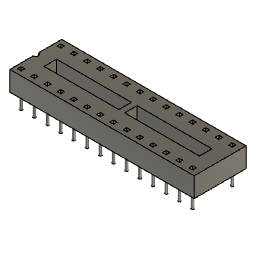
ICSocket_DIP28pin (Autodesk Fusion 360 design; units mm, degrees)
Autodesk Fusion 360 part; units mm, degrees
sketch "スケッチ1" plane through (0, 0, 0) normal (0, 0, 1) x (1, 0, 0)
  line L0 (-17.75, 5) -> (17.75, 5)
  line L1 (17.75, 5) -> (17.75, -5)
  line L2 (17.75, -5) -> (-17.75, -5)
  line L3 (-17.75, -5) -> (-17.75, 5)
  dimension "d1" = 35.5
  dimension "d2" = 10
  dimension "d3" = 17.75
  dimension "d4" = 5
  constraint horizontal L0
  constraint vertical L1
  constraint horizontal L2
  constraint vertical L3
  measures "d1" distance of L0.start L0.end
  measures "d2" distance of L0.start L2.end
  measures "d3" distance of origin L3
  measures "d4" distance of origin L0
extrude "押し出し1" add sketch "スケッチ1" along normal blind 3.8
sketch "スケッチ2" plane through (0, 0, 3.8) normal (0, 0, 1) x (-1, 0, 0)
  line L0 (17.75, 5) -> (-17.75, 5)
  line L1 (-17.75, 5) -> (-17.75, -5)
  line L2 (-17.75, -5) -> (17.75, -5)
  line L3 (17.75, -5) -> (17.75, 5)
  line L4 (-0.55, -1.2) -> (-14.95, -1.2)
  line L5 (-14.95, -1.2) -> (-14.95, 1.2)
  line L6 (-14.95, 1.2) -> (-0.55, 1.2)
  line L7 (-0.55, 1.2) -> (-0.55, -1.2)
  line L8 (14.95, -1.2) -> (0.55, -1.2)
  line L9 (0.55, -1.2) -> (0.55, 1.2)
  line L10 (0.55, 1.2) -> (14.95, 1.2)
  line L11 (14.95, 1.2) -> (14.95, -1.2)
  line L12 (0, -1.75) -> (0, -22.5)
  line L13 (17.11, 3.46) -> (16.41, 3.46)
  line L14 (16.41, 3.46) -> (16.41, 4.16)
  line L15 (16.41, 4.16) -> (17.11, 4.16)
  line L16 (17.11, 4.16) -> (17.11, 3.46)
  arc A0 (17.75, 0.5) -> (17.75, -0.5) centre (17.75, 0) ccw
  line L17 (17.75, 0) -> (17.75, 0.5) construction
  line L18 (17.75, 0) -> (17.75, -0.5) construction
  dimension "d7" = 14.4
  dimension "d8" = 2.4
  dimension "d9" = 3.8
  dimension "d10" = 2.8
  dimension "d11" = 14.4
  dimension "d12" = 2.4
  dimension "d17" = 0.7
  dimension "d18" = 0.7
  dimension "d19" = 3.46
  dimension "d20" = 0.64
  dimension "d38" = 0.5
  dimension "d39" = 180
  constraint horizontal L4
  constraint vertical L5
  constraint horizontal L6
  constraint vertical L7
  constraint horizontal L8
  constraint vertical L9
  constraint horizontal L10
  constraint vertical L11
  constraint collinear L6 L10
  constraint symmetric L7 L9 L12
  constraint horizontal L13
  constraint vertical L14
  constraint horizontal L15
  constraint vertical L16
  constraint midpoint L3 A0.centre
  measures "d7" distance of L4.start L4.end
  measures "d8" distance of L4.start L6.end
  measures "d9" distance of L0 L6
  measures "d10" distance of L1 L5
  measures "d11" distance of L8.start L8.end
  measures "d12" distance of L8.start L10.end
  measures "d17" distance of L13.start L13.end
  measures "d18" distance of L13.start L15.end
  measures "d19" distance of origin L13
  measures "d20" distance of L3 L16
  measures "d38" radius of A0
  measures "d39" angle of L17 L18
extrude "押し出し2" cut sketch "スケッチ2" against normal through all contours L3 A0 | L4 L5 L6 L7 | L8 L9 L10 L11
extrude "押し出し3" cut sketch "スケッチ2" against normal blind 3.5 contours L13 L14 L15 L16
pattern_linear "R パターン1" count 14 spacing 2.54 along (1, 0, 0) of "押し出し3"
mirror "ミラー1" about plane through (0, 0, 0) normal (0, 1, 0) of "押し出し3", "R パターン1"
sketch "スケッチ3" plane through (0, 0, 0) normal (0, 0, -1) x (1, 0, 0)
  line L0 (0.55, -1.2) -> (0.55, 1.2)
  line L1 (0.55, 1.2) -> (14.95, 1.2)
  line L2 (14.95, 1.2) -> (14.95, -1.2)
  line L3 (14.95, -1.2) -> (0.55, -1.2)
  line L4 (-14.95, -1.2) -> (-14.95, 1.2)
  line L5 (-14.95, 1.2) -> (-0.55, 1.2)
  line L6 (-0.55, 1.2) -> (-0.55, -1.2)
  line L7 (-0.55, -1.2) -> (-14.95, -1.2)
  line L8 (17.75, 5) -> (-17.75, 5)
  line L9 (-17.75, -0.5) -> (-17.75, -5)
  line L10 (-17.75, -5) -> (17.75, -5)
  line L11 (17.75, -5) -> (17.75, 5)
  line L12 (-16.41, 4.16) -> (-17.11, 4.16)
  line L13 (-16.41, 3.46) -> (-16.41, 4.16)
  line L14 (-17.11, 3.46) -> (-16.41, 3.46)
  line L15 (-17.11, 4.16) -> (-17.11, 3.46)
  circle A0 centre (-16.76, 3.81) radius 0.25
  arc A1 (-17.75, -0.5) -> (-17.75, 0.5) centre (-17.75, 0) ccw
  line L16 (-17.75, 5) -> (-17.75, 0.5)
  dimension "d28" = 0.5
  dimension "d29" = 0.35
  dimension "d30" = 0.35
  measures "d28" diameter of A0
  measures "d29" distance of L12 A0.centre
  measures "d30" distance of L15 A0.centre
extrude "押し出し4" add sketch "スケッチ3" along normal blind 3 contours A0
pattern_linear "R パターン2" count 14 spacing 2.54 along (1, 0, 0) of "押し出し4"
mirror "ミラー2" about plane through (0, 0, 0) normal (0, 1, 0) of "押し出し4", "R パターン2"
